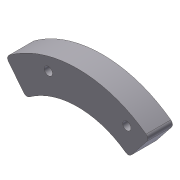
# Autodesk Inventor part: FlyWheel_Weight_Jan21
Saved by Autodesk Inventor 2012 (Build 160160000, 160)
## iProperties
Created: 2012-01-22
Part Number: FlyWheel_Weight_Jan21
Material: Aluminum-6061
Document SubType Name: Modeling
Designer: JesseK
Mass: 127.082 g
Surface Area: 103.48 cm^2
Volume: 46.8936 cm^3
Density: 2.71 g/cm^3
Author: JesseK
Autodesk Inventor part; units mm, degrees
ref_plane "YZ Plane" through (0, 0, 0) normal (1, 0, 0) x (0, 1, 0)
ref_plane "XZ Plane" through (0, 0, 0) normal (0, 1, 0) x (-1, 0, 0)
ref_plane "XY Plane" through (0, 0, 0) normal (0, 0, 1) x (1, 0, 0)
sketch "Sketch1" plane through (0, 0, 0) normal (0, 0, 1) x (1, 0, 0)
  arc A0 (37.1184, 51.5216) -> (-37.1184, 51.5216) centre (0, 0) ccw
  arc A1 (37.8745, 69.7561) -> (-22.5437, 76.1063) centre (0, 0) ccw construction
  arc A2 (52.7268, 71.5758) -> (-52.7268, 71.5758) centre (0, 0) ccw
  circle A3 centre (-22.5437, 76.1063) radius 3.175
  circle A4 centre (37.8745, 69.7561) radius 3.175
  line L0 (37.8745, 69.7561) -> (0, 0) construction
  line L1 (0, 0) -> (-22.5437, 76.1063) construction
  line L2 (0, 79.375) -> (0, 0) construction
  line L3 (-22.5437, 76.1063) -> (0, 79.375) construction
  line L4 (0, 79.375) -> (37.8745, 69.7561) construction
  line L5 (-53.3285, 67.0431) -> (-41.4591, 52.1212)
  line L6 (41.4591, 52.1212) -> (53.3285, 67.0431)
  line L7 (-39.5297, 49.6956) -> (0, 0) construction
  line L8 (0, 0) -> (39.5297, 49.6956) construction
  line L9 (-39.5297, 49.6956) -> (0, 63.5) construction
  line L10 (0, 63.5) -> (39.5297, 49.6956) construction
  arc A5 (-52.7268, 71.5758) -> (-53.3285, 67.0431) centre (-50.8437, 69.0195) ccw
  arc A6 (-41.4591, 52.1212) -> (-37.1184, 51.5216) centre (-38.9743, 54.0977) ccw
  arc A7 (37.1184, 51.5216) -> (41.4591, 52.1212) centre (38.9743, 54.0977) ccw
  arc A8 (53.3285, 67.0431) -> (52.7268, 71.5758) centre (50.8437, 69.0195) ccw
  point P0 (55.3416, 69.5739)
  point P1 (-55.3416, 69.5739)
  dimension "d0" = 79.375
  dimension "d1" = 88.9
  dimension "d2" = 45
  dimension "d5" = 3.175
  dimension "d8" = 6.35
  dimension "d9" = 63.5
  dimension "d10" = 22
  dimension "d11" = 10
  constraints: 22 end point, 20 point on circle, 9 centre point, 8 tangent, 5 coincident, 5 point on line, 4 equal radius, 2 collinear, 1 equal length, 1 vertical
  measures "d0" radius of A1
  measures "d1" radius of A2
  measures "d2" angle of L0 L1
  measures "d5" radius of A5
  measures "d8" diameter of A3
  measures "d9" radius of A0
  measures "d10" angle of L1 L5
  measures "d11" angle of L6 L0
extrude "Extrusion1" add sketch "Sketch1" along normal blind 19.05
body "Solid1"
